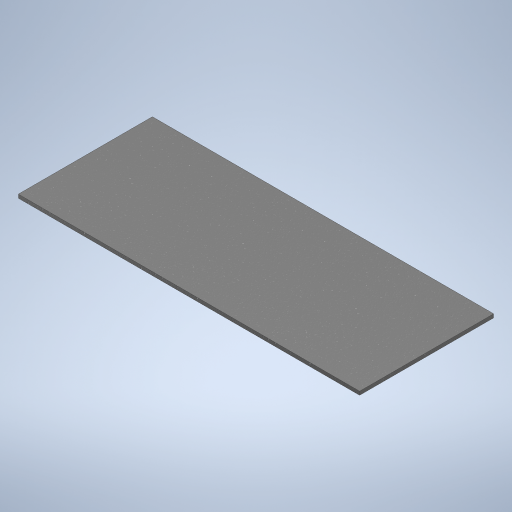
# Autodesk Inventor part: BottomHalfOfBack
Saved by Autodesk Inventor 2023 (Build 270158000, 158)
## iProperties
Created: 2025-03-05
Part Number: BottomHalfOfBack
Material: Generic
Document SubType Name: Modeling
Designer: FrameUser
Density: 1 g/cm^3
Appearance: Default
Author: FrameUser
Autodesk Inventor part; units mm, degrees
ref_plane "YZ Plane" through (0, 0, 0) normal (1, 0, 0) x (0, 1, 0)
ref_plane "XZ Plane" through (0, 0, 0) normal (0, 1, 0) x (-1, 0, 0)
ref_plane "XY Plane" through (0, 0, 0) normal (0, 0, 1) x (1, 0, 0)
sketch "Sketch1" plane through (0, 0, 0) normal (0, 1, 0) x (-1, 0, 0)
  line L0 (0, 0) -> (-614.3625, 0)
  line L1 (-614.3625, 0) -> (-614.3625, -228.6)
  line L2 (-614.3625, -228.6) -> (0, -228.6)
  line L3 (0, -228.6) -> (0, 0)
  dimension "d0" = 614.3625
  dimension "d1" = 228.6
  constraints: 8 end point, 2 perpendicular, 1 horizontal, 1 vertical
  measures "d0" distance of L0.start L0.end
  measures "d1" distance of L0.end L1.end
extrude "Extrusion1" add sketch "Sketch1" along normal blind 6.35
sketch "Sketch2" plane through (0, 6.35, 0) normal (0, 1, 0) x (1, 0, 0)
  line L0 (614.3625, 228.6) -> (0, 228.6) projected
  line L1 (0, 228.6) -> (0, 241.3)
  line L2 (0, 241.3) -> (614.3625, 241.3)
  line L3 (614.3625, 241.3) -> (614.3625, 228.6)
  line L4 (614.3625, 228.6) -> (0, 228.6)
  point P0 (0, 0)
  dimension "d4" = 12.7
  constraints: 8 end point, 2 perpendicular, 1 parallel, 1 vertical
  measures "d4" distance of L0.end L1.end
extrude "Extrusion2" add sketch "Sketch2" against normal blind 6.35
body "Solid1"
